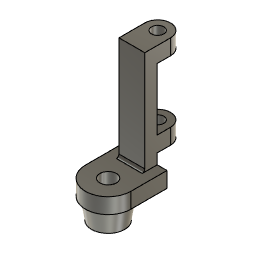
NCV-18 v2 (Autodesk Fusion 360 design; units mm, degrees)
Autodesk Fusion 360 part; units mm, degrees
sketch "Sketch1" plane through (0, 0, 0) normal (0, 0, 1) x (1, 0, 0)
  line L0 (12.5, 0) -> (12.5, -12)
  line L1 (12.5, -12) -> (-12.5, -12)
  line L2 (-12.5, -12) -> (-12.5, 0)
  line L3 (22, 0) -> (22, -35)
  line L4 (-22, -35) -> (-22, 0)
  line L5 (-22, 0) -> (-12.5, 0)
  line L6 (12.5, 0) -> (22, 0)
  circle A0 centre (0, -35) radius 8
  arc A1 (-22, -35) -> (22, -35) centre (0, -35) ccw
  line L7 (-12.5, 0) -> (-12.5, 13)
  circle A2 centre (0, 13) radius 6
  line L8 (12.5, 0) -> (12.5, 13)
  arc A3 (12.5, 13) -> (-12.5, 13) centre (0, 13) ccw
  circle A4 centre (0, -35) radius 19 construction
  circle A5 centre (0, -35) radius 16 construction
  dimension "d1" = 22
  dimension "d2" = 22
  dimension "d3" = 12.5
  dimension "d4" = 12.5
  dimension "d6" = 12
  dimension "d8" = 16
  dimension "d9" = 22
  dimension "d10" = 44
  dimension "d11" = 22
  dimension "d12" = 35
  dimension "d13" = 35
  dimension "d14" = 12
  dimension "d15" = 13
  dimension "d16" = 12
  dimension "d17" = 13
  dimension "d18" = 13
  dimension "d19" = 12.5
  dimension "d20" = 25
  dimension "d21" = 12.5
  dimension "d22" = 13
  dimension "d23" = 38
  dimension "d24" = 32
  constraint vertical L0
  constraint horizontal L1
  constraint vertical L2
  constraint horizontal L5
  constraint vertical L3
  constraint vertical L4
  constraint collinear L5 L6
  constraint perpendicular L5 L7
  constraint perpendicular L6 L8
  constraint concentric A1 A4
  constraint concentric A4 A5
  measures "d1" distance of origin L4
  measures "d2" distance of origin L3
  measures "d3" distance of origin L0
  measures "d4" distance of origin L2
  measures "d6" distance of origin L1
  measures "d8" diameter of A0
  measures "d9" distance of L3 A0.centre
  measures "d10" diameter of A1
  measures "d11" distance of L3 A0.centre
  measures "d12" vertical distance of origin L3.end
  measures "d13" distance of origin A0.centre
  measures "d14" distance of L1 L5
  measures "d15" distance of L2.end L7.end
  measures "d16" diameter of A2
  measures "d17" distance of L0.start L8.end
  measures "d18" vertical distance of origin A2.centre
  measures "d19" distance of L7 A2.centre
  measures "d20" diameter of A3
  measures "d21" distance of L7 A2.centre
  measures "d22" distance of origin A2.centre
  measures "d23" diameter of A4
  measures "d24" diameter of A5
sketch "Sketch2" plane through (0, 0, 0) normal (1, 0, 0) x (0, 1, 0)
  line L0 (0, 0) -> (25.5, 0)
  line L1 (25.5, 0) -> (25.5, 25)
  line L2 (25.5, 25) -> (0, 25)
  line L3 (0, 25) -> (0, 0)
  line L4 (0, 40) -> (25.5, 40)
  line L5 (25.5, 40) -> (25.5, 100)
  line L6 (25.5, 100) -> (0, 100)
  line L7 (0, 100) -> (0, 40)
  line L8 (-12, 17.5) -> (-12, 15)
  line L9 (-12, 15) -> (-14.5, 15)
  arc A0 (-14.5, 15) -> (-12, 17.5) centre (-14.5, 17.5) ccw
  line L10 (-27, 0) -> (-16, 0)
  line L11 (-16, 0) -> (-19, -20)
  line L12 (-19, -20) -> (-27, -20)
  line L13 (-27, -20) -> (-27, 0)
  dimension "d29" = 25.5
  dimension "d30" = 25
  dimension "d31" = 25.5
  dimension "d32" = 25.5
  dimension "d33" = 40
  dimension "d34" = 100
  dimension "d35" = 5
  dimension "d36" = 12
  dimension "d37" = 15
  dimension "d45" = 16
  dimension "d46" = 27
  dimension "d47" = 20
  dimension "d48" = 20
  dimension "d49" = 19
  constraint horizontal L0
  constraint vertical L1
  constraint horizontal L2
  constraint vertical L3
  constraint coincident L0.start L3.end
  constraint horizontal L4
  constraint vertical L5
  constraint horizontal L6
  constraint vertical L7
  constraint vertical L8
  constraint horizontal L9
  constraint tangent L8 A0
  constraint tangent L9 A0
  constraint horizontal L10
  constraint vertical L13
  constraint horizontal L12
  measures "d29" distance of L0.start L1
  measures "d30" distance of L2 L0.start
  measures "d31" distance of L0.start L5
  measures "d32" distance of L5 L7
  measures "d33" distance of L0.start L4
  measures "d34" distance of L0.start L6
  measures "d35" diameter of A0
  measures "d36" horizontal distance of L0.start L8.end
  measures "d37" vertical distance of L0.start L8.end
  measures "d45" distance of L0.start L10.end
  measures "d46" distance of L0.start L10.start
  measures "d47" distance of L0.start L12
  measures "d48" distance of L10 L12
  measures "d49" horizontal distance of L0.start L11.end
extrude "Extrude1" add sketch "Sketch1" along normal blind 15 contours L0 L1 L2 L3 L4 L5 L6 A1
extrude "Extrude2" add sketch "Sketch1" along normal blind 115 contours L0 L1 L2 L7 L8 A3
extrude "Extrude3" add sketch "Sketch2" along normal up to surface (-25 mm away) and the other way blind 0 from surface at 12.5 contours L8 L9 A0
extrude "Extrude4" cut sketch "Sketch2" along normal through all and the other way through all contours L0 L1 L2 L3 | L4 L5 L6 L7
revolve "Revolve1" add sketch "Sketch2" angle 360 about axis through (0, -35, 0) along (0, 0, -1) contours L10 L11 L12 L13
equation "d19 = d4"
equation "d21 = d19"
equation "d22 = d18"
equation "d31 = d29"
equation "d32 = d31"
equation "d33 = d30 + 15 mm"
equation "d34 = d33 + 60 mm"
equation "d45 = 35 mm - ( 38 / 2 ) * 1 mm"
equation "d46 = 35 mm - ( 16 / 2 ) * 1 mm"
equation "d49 = 35 mm - ( 32 / 2 ) * 1 mm"
